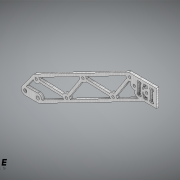
# Autodesk Inventor part: 横回転カウンター根本
Saved by Autodesk Inventor 2020 (Build 240168000, 168)
## iProperties
Created: 2020-02-27
Part Number: 横回転カウンター根本
Material: アルミニウム 7075
Document SubType Name: Modeling
Designer: tanjihayato
Density: 2.81 g/cm^3
Appearance: サテン - ブラシ仕上げ 重厚
Author: tanjihayato
Autodesk Inventor part; units mm, degrees
ref_plane "YZ Plane" through (0, 0, 0) normal (1, 0, 0) x (0, 1, 0)
ref_plane "XZ Plane" through (0, 0, 0) normal (0, 1, 0) x (-1, 0, 0)
ref_plane "XY Plane" through (0, 0, 0) normal (0, 0, 1) x (1, 0, 0)
sketch "スケッチ1" plane through (0, 0, 0) normal (0, 0, 1) x (1, 0, 0)
  line L0 (0, 0) -> (3, 0)
  line L1 (3, 0) -> (3, -15)
  line L2 (3, -15) -> (0, -15)
  line L3 (0, -15) -> (0, 0)
  line L4 (-15, 0) -> (-12, 0)
  line L5 (-12, 0) -> (-12, -15)
  line L6 (-12, -15) -> (-15, -15)
  line L7 (-15, -15) -> (-15, 0)
  line L8 (-26.0926, 3) -> (-139.0635, -55.2952)
  line L9 (7, 3) -> (7, -18)
  line L10 (-7.8217, -18) -> (-133.786, -83)
  circle A0 centre (-135, -78) radius 2
  circle A1 centre (-150, -78) radius 2
  line L11 (-150, -78) -> (-135, -78) construction
  arc A2 (-154.0422, -75.0571) -> (-150, -83) centre (-150, -78) ccw
  line L12 (-140.638, -56.6456) -> (-154.0422, -75.0571)
  circle A3 centre (-15, -1.05) radius 1.05
  circle A4 centre (-15, -13.95) radius 1.05
  circle A5 centre (-12, -13.95) radius 1.05
  circle A6 centre (-12, -1.05) radius 1.05
  circle A7 centre (0, -1.05) radius 1.05
  circle A8 centre (3, -1.05) radius 1.05
  circle A9 centre (0, -13.95) radius 1.05
  circle A10 centre (3, -13.95) radius 1.05
  arc A11 (-139.0635, -55.2952) -> (-140.638, -56.6456) centre (-137, -59.2941) ccw
  circle A12 centre (-100.7273, -60.8773) radius 4.5 construction
  circle A13 centre (-81, -30.3971) radius 4.5 construction
  circle A14 centre (-44.7273, -31.9802) radius 4.5 construction
  circle A15 centre (-25, -1.5) radius 4.5 construction
  circle A16 centre (-137, -59.2941) radius 1.5
  circle A17 centre (-100.7273, -60.8773) radius 1.5
  circle A18 centre (-81, -30.3971) radius 1.5
  circle A19 centre (-44.7273, -31.9802) radius 1.5
  circle A20 centre (-25, -1.5) radius 1.5
  circle A21 centre (-4.5, -7.5) radius 1.5
  circle A22 centre (-19.5, -7.5) radius 1.5
  line L13 (-26.0926, 3) -> (7, 3)
  line L14 (-7.8217, -18) -> (7, -18)
  line L15 (-150, -83) -> (-133.786, -83)
  circle A23 centre (-135, -78) radius 5
  line L16 (-25, -1.5) -> (-44.7273, -31.9802) construction
  line L17 (-44.7273, -31.9802) -> (-81, -30.3971) construction
  line L18 (-81, -30.3971) -> (-100.7273, -60.8773) construction
  line L19 (-100.7273, -60.8773) -> (-137, -59.2941) construction
  point P0 (0, -12.9)
  point P1 (0, -2.1)
  point P2 (3, -2.1)
  point P3 (3, -12.9)
  point P4 (-12, -2.1)
  point P5 (-12, -12.9)
  point P6 (-15, -12.9)
  point P7 (-15, -2.1)
  dimension "d0" = 3
  dimension "d1" = 15
  dimension "d2" = 3
  dimension "d3" = 15
  dimension "d4" = 12
  dimension "d5" = 4
  dimension "d6" = 4
  dimension "d7" = 15
  dimension "d8" = 4
  dimension "d12" = 3
  dimension "d13" = 2.1
  dimension "d14" = 2.1
  dimension "d15" = 2.1
  dimension "d16" = 2.1
  dimension "d17" = 2.1
  dimension "d18" = 2.1
  dimension "d19" = 2.1
  dimension "d20" = 2.1
  dimension "d23" = 9
  dimension "d24" = 9
  dimension "d25" = 9
  dimension "d26" = 9
  dimension "d27" = 9
  dimension "d28" = 3
  dimension "d29" = 3
  dimension "d30" = 3
  dimension "d31" = 3
  dimension "d32" = 3
  dimension "d33" = 10
  dimension "d34" = 3
  dimension "d35" = 3
  dimension "d36" = 4.5
  dimension "d37" = 4.5
  dimension "d38" = 7.5
  dimension "d39" = 7.5
  dimension "d60" = 120
  dimension "d61" = 3
  dimension "d62" = 3
  dimension "d63" = 3
  dimension "d64" = 60
  constraints: 40 end point, 24 centre point, 18 tangent, 8 point on line, 7 parallel, 6 horizontal, 5 coincident, 4 point on circle, 2 perpendicular, 1 collinear, 1 equal length, 1 vertical
  measures "d0" distance of L1.end L2.end
  measures "d1" distance of L0.end L1.end
  measures "d2" distance of L5.end L6.end
  measures "d3" distance of L4.end L5.end
  measures "d4" distance between parallel lines of L5 L3
  measures "d5" diameter of A0
  measures "d6" diameter of A1
  measures "d7" distance of L11.start L11.end
  measures "d8" distance between parallel lines of L9 L1
  measures "d12" radial gap between concentric circles of A1 A2
  measures "d13" diameter of A3
  measures "d14" diameter of A4
  measures "d15" diameter of A5
  measures "d16" diameter of A6
  measures "d17" diameter of A7
  measures "d18" diameter of A8
  measures "d19" diameter of A9
  measures "d20" diameter of A10
  measures "d23" diameter of A11
  measures "d24" diameter of A12
  measures "d25" diameter of A13
  measures "d26" diameter of A14
  measures "d27" diameter of A15
  measures "d28" diameter of A16
  measures "d29" diameter of A17
  measures "d30" diameter of A18
  measures "d31" diameter of A19
  measures "d32" diameter of A20
  measures "d33" distance from line of A15.centre L7
  measures "d34" diameter of A21
  measures "d35" diameter of A22
  measures "d36" distance from line of A22.centre L7
  measures "d37" distance from line of L3 A21.centre
  measures "d38" distance from line of A22.centre L4
  measures "d39" distance from line of L0 A21.centre
  measures "d60" distance from line of L11.end L7
  measures "d61" radial gap between concentric circles of A0 A23
  measures "d62" distance between parallel lines of L13 L0
  measures "d63" distance between parallel lines of L14 L2
  measures "d64" distance between parallel lines of L11 L14
extrude "押し出し1" add sketch "スケッチ1" along normal blind 3
sketch "スケッチ3" plane through (0, 0, 3) normal (0, 0, 1) x (1, 0, 0)
  line L0 (-150, -83) -> (-133.786, -83) projected
  line L1 (-133.786, -83) -> (-7.8217, -18) projected
  line L2 (-7.8217, -18) -> (7, -18) projected
  line L3 (7, -18) -> (7, 3) projected
  line L4 (7, 3) -> (-26.0926, 3) projected
  line L5 (-26.0926, 3) -> (-139.0635, -55.2952) projected
  arc A0 (-139.0635, -55.2952) -> (-140.638, -56.6456) centre (-137, -59.2941) ccw projected
  line L6 (-140.638, -56.6456) -> (-154.0422, -75.0571) projected
  arc A1 (-154.0422, -75.0571) -> (-150, -83) centre (-150, -78) ccw projected
  circle A2 centre (-19.5, -7.5) radius 1.5 projected
  circle A3 centre (-25, -1.5) radius 1.5 projected
  circle A4 centre (-44.7273, -31.9802) radius 1.5 projected
  circle A5 centre (-81, -30.3971) radius 1.5 projected
  circle A6 centre (-100.7273, -60.8773) radius 1.5 projected
  circle A7 centre (-137, -59.2941) radius 1.5 projected
  arc A8 (3, -2.1) -> (3, 0) centre (3, -1.05) ccw projected
  line L7 (3, -2.1) -> (3, -12.9) projected
  arc A9 (3, -15) -> (3, -12.9) centre (3, -13.95) ccw projected
  line L8 (3, -15) -> (0, -15) projected
  arc A10 (0, -12.9) -> (0, -15) centre (0, -13.95) ccw projected
  line L9 (0, -12.9) -> (0, -2.1) projected
  arc A11 (0, 0) -> (0, -2.1) centre (0, -1.05) ccw projected
  line L10 (0, 0) -> (3, 0) projected
  circle A12 centre (-135, -78) radius 2 projected
  line L11 (-12, -2.1) -> (-12, -12.9) projected
  arc A13 (-12, -15) -> (-12, -12.9) centre (-12, -13.95) ccw projected
  line L12 (-12, -15) -> (-15, -15) projected
  arc A14 (-15, -12.9) -> (-15, -15) centre (-15, -13.95) ccw projected
  line L13 (-15, -12.9) -> (-15, -2.1) projected
  arc A15 (-15, 0) -> (-15, -2.1) centre (-15, -1.05) ccw projected
  line L14 (-15, 0) -> (-12, 0) projected
  arc A16 (-12, -2.1) -> (-12, 0) centre (-12, -1.05) ccw projected
  circle A17 centre (-4.5, -7.5) radius 1.5 projected
  circle A18 centre (-150, -78) radius 2 projected
  line L15 (-137.6878, -57.9612) -> (-25.3642, 0)
  line L16 (-25.3642, 0) -> (4, 0)
  line L17 (4, 0) -> (4, -15)
  line L18 (4, -15) -> (-8.5501, -15)
  line L19 (-8.5501, -15) -> (-134.5144, -80)
  line L20 (-134.5144, -80) -> (-150, -80)
  arc A19 (-151.6169, -76.8229) -> (-150, -80) centre (-150, -78) ccw
  line L21 (-151.6169, -76.8229) -> (-138.2127, -58.4113)
  arc A20 (-137.6878, -57.9612) -> (-138.2127, -58.4113) centre (-137, -59.2941) ccw
  circle A21 centre (-81, -30.3971) radius 4.5
  circle A22 centre (-100.7273, -60.8773) radius 4.5
  circle A23 centre (-137, -59.2941) radius 4.5
  circle A24 centre (-44.7273, -31.9802) radius 4.5
  circle A25 centre (-19.5, -7.5) radius 4.5
  line L22 (-9, -11.2292) -> (-9, -3.7708)
  arc A26 (-9, -3.7708) -> (-12, 3) centre (-12, -1.05) ccw
  line L23 (-12, 3) -> (-15, 3)
  arc A27 (-15, 3) -> (-18, -3.7708) centre (-15, -1.05) ccw
  line L24 (-18, -3.7708) -> (-18, -11.2292)
  arc A28 (-18, -11.2292) -> (-15, -18) centre (-15, -13.95) ccw
  line L25 (-15, -18) -> (-12, -18)
  arc A29 (-12, -18) -> (-9, -11.2292) centre (-12, -13.95) ccw
  circle A30 centre (-25, -1.5) radius 4.5
  line L26 (-3, -3.7708) -> (-3, -11.2292)
  arc A31 (-3, -11.2292) -> (0, -18) centre (0, -13.95) ccw
  line L27 (0, -18) -> (3, -18)
  arc A32 (3, -18) -> (6, -11.2292) centre (3, -13.95) ccw
  line L28 (6, -11.2292) -> (6, -3.7708)
  arc A33 (6, -3.7708) -> (3, 3) centre (3, -1.05) ccw
  line L29 (3, 3) -> (0, 3)
  arc A34 (0, 3) -> (-3, -3.7708) centre (0, -1.05) ccw
  circle A35 centre (-4.5, -7.5) radius 4.6
  circle A36 centre (-135, -78) radius 5
  circle A37 centre (-150, -78) radius 5
  line L30 (-135, -73) -> (-150, -73)
  circle A38 centre (-137, -59.2941) radius 1.5 projected
  line L31 (-137, -59.2941) -> (-100.7273, -60.8773) construction
  line L32 (-137.0654, -60.7927) -> (-100.7927, -62.3759)
  line L33 (-100.6619, -59.3787) -> (-136.9346, -57.7956)
  arc A39 (-136.9346, -57.7956) -> (-137.0654, -60.7927) centre (-137, -59.2941) ccw
  arc A40 (-100.7927, -62.3759) -> (-100.6619, -59.3787) centre (-100.7273, -60.8773) ccw
  line L34 (-81, -30.3971) -> (-100.7273, -60.8773) construction
  line L35 (-82.2593, -29.5821) -> (-101.9866, -60.0623)
  line L36 (-99.4681, -61.6923) -> (-79.7407, -31.2121)
  arc A41 (-79.7407, -31.2121) -> (-82.2593, -29.5821) centre (-81, -30.3971) ccw
  arc A42 (-101.9866, -60.0623) -> (-99.4681, -61.6923) centre (-100.7273, -60.8773) ccw
  line L37 (-81, -30.3971) -> (-44.7273, -31.9802) construction
  line L38 (-81.0654, -31.8956) -> (-44.7927, -33.4788)
  line L39 (-44.6619, -30.4816) -> (-80.9346, -28.8985)
  arc A43 (-80.9346, -28.8985) -> (-81.0654, -31.8956) centre (-81, -30.3971) ccw
  arc A44 (-44.7927, -33.4788) -> (-44.6619, -30.4816) centre (-44.7273, -31.9802) ccw
  line L40 (-25, -1.5) -> (-44.7273, -31.9802) construction
  line L41 (-26.2593, -0.685) -> (-45.9866, -31.1652)
  line L42 (-43.4681, -32.7952) -> (-23.7407, -2.315)
  arc A45 (-23.7407, -2.315) -> (-26.2593, -0.685) centre (-25, -1.5) ccw
  arc A46 (-45.9866, -31.1652) -> (-43.4681, -32.7952) centre (-44.7273, -31.9802) ccw
  point P0 (-118.8637, -60.0857)
  point P1 (-90.8637, -45.6372)
  point P2 (-62.8637, -31.1886)
  point P3 (-34.8637, -16.7401)
  point P4 (-3.5501, -12.0009)
  point P5 (-9, -8.4539)
  point P6 (-8.0885, -15)
  point P7 (-3.9115, -15)
  point P8 (-9, -6.5461)
  point P9 (-3.5501, -2.9991)
  point P10 (-3.9115, 0)
  point P11 (-8.0885, 0)
  point P12 (-26.046, -5.8768)
  point P13 (-41.1629, -29.2335)
  point P14 (-40.2692, -31.3677)
  point P15 (-14.3638, -18)
  point P16 (-18.4832, -11.8836)
  point P17 (-23.6655, -5.7976)
  point P18 (-43.6814, -27.6035)
  point P19 (-28.5645, -4.2467)
  point P20 (-29.4581, -2.1125)
  point P21 (-77.9176, -27.1186)
  point P22 (-76.696, -29.0835)
  point P23 (-48.9005, -30.2967)
  point P24 (-49.0314, -33.2938)
  point P25 (-76.8268, -32.0806)
  point P26 (-82.046, -34.7738)
  point P27 (-97.1629, -58.1306)
  point P28 (-96.2692, -60.2648)
  point P29 (-47.8098, -35.2587)
  point P30 (-99.6814, -56.5005)
  point P31 (-84.5645, -33.1438)
  point P32 (-85.4581, -31.0096)
  point P33 (-133.9176, -56.0156)
  point P34 (-132.696, -57.9806)
  point P35 (-104.9005, -59.1937)
  point P36 (-105.0314, -62.1909)
  point P37 (-132.8268, -60.9777)
  point P38 (-140.7098, -61.8412)
  point P39 (-148.8337, -73)
  point P40 (-130.0105, -77.6759)
  point P41 (-103.8098, -64.1558)
  dimension "d65" = 3
  dimension "d66" = 3
  dimension "d67" = 3
  dimension "d68" = 3
  dimension "d69" = 3
  dimension "d70" = 3
  dimension "d71" = 3
  dimension "d72" = 3
  dimension "d73" = 3
  dimension "d74" = 3.1
  dimension "d75" = 3
  dimension "d76" = 3
  dimension "d77" = 3
  dimension "d78" = 3
  dimension "d79" = 3
  dimension "d80" = 3
  constraints: 64 end point, 36 point on circle, 25 centre point, 16 tangent, 5 parallel, 4 concentric, 4 midpoint, 2 horizontal, 1 vertical alignment, 27 other
  measures "d65" distance between parallel lines of L5 L15
  measures "d66" radial gap between concentric circles of A5 A21
  measures "d67" radial gap between concentric circles of A6 A22
  measures "d68" radial gap between concentric circles of A7 A23
  measures "d69" radial gap between concentric circles of A4 A24
  measures "d70" radial gap between concentric circles of A2 A25
  measures "d71" radial gap between concentric circles of A13 A29
  measures "d72" radial gap between concentric circles of A3 A30
  measures "d73" distance between parallel lines of L9 L26
  measures "d74" radial gap between concentric circles of A17 A35
  measures "d77" diameter of A40
  measures "d78" diameter of A42
  measures "d79" diameter of A44
  measures "d80" diameter of A46
extrude "押し出し3" cut sketch "スケッチ3" against normal blind 3 contours L30 L21 A23 L32 A22 L19 A36 | L15 A21 L35 A22 L33 A23 | L19 A22 L36 A21 L38 A24 | L15 A30 L41 A24 L39 A21 | A24 L42 A30 A25 A28 L25 L19 | L18 A29 L22 A35 A31 | L16 A34 A35 L22 A26
